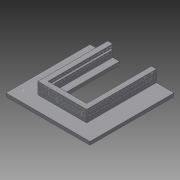
# Autodesk Inventor part: Halterung Merkruphy
Saved by Autodesk Inventor 2015 (Build 190159000, 159)
## iProperties
Created: 2017-01-12
Part Number: Halterung Merkruphy
Material: Generisch
Document SubType Name: Modeling
Designer: nikla
Density: 1 g/cm^3
Appearance: Vorgabe
Author: nikla
Autodesk Inventor part; units mm, degrees
ref_plane "YZ Plane" through (0, 0, 0) normal (1, 0, 0) x (0, 1, 0)
ref_plane "XZ Plane" through (0, 0, 0) normal (0, 1, 0) x (-1, 0, 0)
ref_plane "XY Plane" through (0, 0, 0) normal (0, 0, 1) x (1, 0, 0)
sketch "Skizze4" plane through (0, 0, 0) normal (0, 0, 1) x (1, 0, 0)
  line L0 (0, 0) -> (50, 0)
  line L1 (50, 0) -> (50, 50)
  line L2 (50, 50) -> (0, 50)
  line L3 (0, 50) -> (0, 0)
  dimension "d5" = 50
  dimension "d6" = 50
  constraints: 8 end point, 2 parallel, 1 horizontal, 1 perpendicular
  measures "d5" distance of L2.end L1.end
  measures "d6" distance of L1.end L0.end
extrude "Extrusion1" add sketch "Skizze4" along normal blind 2
sketch "Skizze5" plane through (0, 0, 2) normal (0, 0, 1) x (1, 0, 0)
  line L0 (50, 50) -> (0, 50) projected
  line L1 (17.5, 50) -> (32.5, 50)
  line L2 (32.5, 50) -> (32.5, 12.5)
  line L3 (32.5, 12.5) -> (17.5, 12.5)
  line L4 (17.5, 12.5) -> (17.5, 50)
  point P0 (0, 0)
  dimension "d10" = 15
  dimension "d11" = 37.5
  constraints: 8 end point, 2 parallel, 1 horizontal, 1 perpendicular, 1 point on line
  measures "d10" distance of L2.end L3.end
  measures "d11" distance of L1.end L2.end
extrude "Extrusion2" cut sketch "Skizze5" against normal blind 2
sketch "Skizze6" plane through (0, 0, 2) normal (0, 0, 1) x (1, 0, 0)
  line L0 (17.5, 50) -> (0, 50) projected
  line L1 (12.5, 50) -> (10.5, 50)
  line L2 (10.5, 50) -> (10.5, 10.5)
  line L3 (10.5, 10.5) -> (12.5, 10.5)
  line L4 (12.5, 12.5) -> (12.5, 50)
  line L5 (10.5, 10.5) -> (39.5, 10.5)
  line L6 (39.5, 10.5) -> (39.5, 12.5)
  line L7 (37.5, 12.5) -> (12.5, 12.5)
  line L8 (10.5, 12.5) -> (10.5, 10.5)
  line L9 (50, 50) -> (32.5, 50) projected
  line L10 (39.5, 10.5) -> (37.5, 10.5)
  line L11 (37.5, 12.5) -> (37.5, 50)
  line L12 (37.5, 50) -> (39.5, 50)
  line L13 (39.5, 50) -> (39.5, 10.5)
  point P0 (0, 0)
  dimension "d14" = 2
  dimension "d15" = 39.5
  dimension "d16" = 29
  dimension "d17" = 2
  dimension "d18" = 2
  constraints: 24 end point, 6 parallel, 3 horizontal, 3 perpendicular, 2 point on line
  measures "d14" distance of L3.end L2.end
  measures "d15" distance of L2.end L1.end
  measures "d16" distance of L8.start L6.end
  measures "d17" distance of L6.end L5.end
  measures "d18" distance of L11.end L12.end
extrude "Extrusion3" add sketch "Skizze6" along normal blind 9
sketch "Skizze7" plane through (37.5, 12.5, 2) normal (-1, 0, 0) x (0, 0, 1)
  line L0 (0, -12.5) -> (0, 37.5) projected
  line L1 (9, 37.5) -> (0, 37.5)
  line L2 (0, 37.5) -> (0, 0)
  line L3 (0, 0) -> (9, 0)
  line L4 (9, 0) -> (9, 37.5)
  point P0 (-2, -12.5)
  dimension "d21" = 37.5
  constraints: 8 end point, 2 parallel, 1 horizontal, 1 perpendicular, 1 point on line
  measures "d21" distance of L2.end L1.end
extrude "Extrusion4" add sketch "Skizze7" along normal blind 2
sketch "Skizze9" plane through (35.5, 12.5, 2) normal (-1, 0, 0) x (0, 0, 1)
  line L0 (9, 0) -> (0, 0) projected
  line L1 (7, 37.5) -> (6, 37.5)
  line L2 (6, 37.5) -> (6, 0)
  line L3 (6, 0) -> (7, 0)
  line L4 (7, 0) -> (7, 37.5)
  point P0 (-2, -12.5)
  dimension "d24" = 1
  constraints: 8 end point, 2 parallel, 1 horizontal, 1 perpendicular, 1 point on line
  measures "d24" distance of L3.end L2.end
extrude "Extrusion5" cut sketch "Skizze9" against normal blind 1
sketch "Skizze10" plane through (17.5, 12.5, 0) normal (0, 1, 0) x (1, 0, 0)
  line L0 (18, -2) -> (-5, -2)
  line L1 (-5, -2) -> (-5, -11)
  line L2 (-5, -11) -> (18, -11)
  line L3 (18, -11) -> (18, -2)
  point P0 (-17.5, 0)
  constraints: 8 end point, 2 parallel, 1 horizontal, 1 perpendicular
extrude "Extrusion6" add sketch "Skizze10" along normal blind 2
sketch "Skizze11" plane through (17.5, 14.5, 0) normal (0, 1, 0) x (1, 0, 0)
  line L0 (-5, -11) -> (-5, -2) projected
  line L1 (19, -9) -> (-5, -9)
  line L2 (-5, -9) -> (-5, -8)
  line L3 (-5, -8) -> (19, -8)
  line L4 (19, -8) -> (19, -9)
  point P0 (-17.5, 0)
  constraints: 8 end point, 2 parallel, 1 horizontal, 1 perpendicular, 1 point on line
extrude "Extrusion7" cut sketch "Skizze11" against normal blind 1
sketch "Skizze12" plane through (36.5, 12.5, 9) normal (0, 1, 0) x (1, 0, 0)
  line L0 (-1, 1) -> (0, 1)
  line L1 (0, 1) -> (0, 0)
  line L2 (0, 0) -> (-1, 0)
  line L3 (-1, 0) -> (-1, 1)
  point P0 (-36.5, 9)
  constraints: 8 end point, 2 parallel, 1 horizontal, 1 perpendicular
extrude "Extrusion8" add sketch "Skizze12" along normal blind 1
sketch "Skizze13" plane through (12.5, 50, 11) normal (1, 0, 0) x (0, 0, -1)
  line L0 (9, -35.5) -> (9, -37.5) projected
  line L1 (0, 0) -> (9, 0)
  line L2 (9, 0) -> (9, -36.5)
  line L3 (9, -36.5) -> (0, -36.5)
  line L4 (0, -36.5) -> (0, 0)
  point P0 (11, -50)
  constraints: 8 end point, 2 parallel, 1 horizontal, 1 midpoint, 1 perpendicular
extrude "Extrusion9" add sketch "Skizze13" along normal blind 2
sketch "Skizze14" plane through (14.5, 50, 11) normal (1, 0, 0) x (0, 0, -1)
  line L0 (9, 0) -> (0, 0) projected
  line L1 (2, 0) -> (3, 0)
  line L2 (3, 0) -> (3, -37.5)
  line L3 (3, -37.5) -> (2, -37.5)
  line L4 (2, -37.5) -> (2, 0)
  point P0 (11, -50)
  dimension "d35" = 1
  dimension "d36" = 37.5
  constraints: 8 end point, 2 parallel, 1 horizontal, 1 perpendicular, 1 point on line
  measures "d35" distance of L2.end L3.end
  measures "d36" distance of L1.end L2.end
extrude "Extrusion10" cut sketch "Skizze14" against normal blind 1
sketch "Skizze15" plane through (10.5, 10.5, 2) normal (0, -1, 0) x (1, 0, 0)
  line L0 (0, 9) -> (29, 9)
  line L1 (29, 9) -> (29, 0)
  line L2 (29, 0) -> (0, 0)
  line L3 (0, 0) -> (0, 9)
  point P0 (-10.5, -2)
  constraints: 8 end point, 2 parallel, 1 horizontal, 1 perpendicular
extrude "Extrusion11" add sketch "Skizze15" along normal blind 2
sketch "Skizze16" plane through (17.5, 14.5, 0) normal (0, 1, 0) x (1, 0, 0)
  line L0 (-3, -2) -> (18, -2)
  line L1 (18, -2) -> (18, -8)
  line L2 (18, -8) -> (-3, -8)
  line L3 (-3, -8) -> (-3, -2)
  point P0 (-17.5, 0)
  constraints: 8 end point, 2 parallel, 1 horizontal, 1 perpendicular
extrude "Extrusion12" cut sketch "Skizze16" against normal blind 4
sketch "Skizze17" plane through (17.5, 13.5, 0) normal (0, 1, 0) x (1, 0, 0)
  line L0 (-3, -8) -> (19, -8)
  line L1 (19, -8) -> (19, -9)
  line L2 (19, -9) -> (-3, -9)
  line L3 (-3, -9) -> (-3, -8)
  point P0 (-17.5, 0)
  constraints: 8 end point, 2 parallel, 1 horizontal, 1 perpendicular
extrude "Extrusion13" cut sketch "Skizze17" against normal blind 2
sketch "Skizze18" plane through (14.5, 12.5, 9) normal (0, 1, 0) x (1, 0, 0)
  line L0 (0, 1) -> (-1, 1)
  line L1 (-1, 1) -> (-1, 0)
  line L2 (-1, 0) -> (0, 0)
  line L3 (0, 0) -> (0, 1)
  point P0 (-14.5, 9)
  constraints: 8 end point, 2 parallel, 1 horizontal, 1 perpendicular
extrude "Extrusion14" cut sketch "Skizze18" against normal blind 2
sketch "Skizze19" plane through (17.5, 11.5, 0) normal (0, 1, 0) x (1, 0, 0)
  line L0 (-3, -8) -> (19, -8)
  line L1 (19, -8) -> (19, -9)
  line L2 (19, -9) -> (-3, -9)
  line L3 (-3, -9) -> (-3, -8)
  point P0 (-17.5, 0)
  constraints: 8 end point, 2 parallel, 1 horizontal, 1 perpendicular
extrude "Extrusion15" cut sketch "Skizze19" against normal blind 1
sketch "Skizze20" plane through (36.5, 12.5, 2) normal (-1, 0, 0) x (0, 0, 1)
  line L0 (6, 37.5) -> (7, 37.5)
  line L1 (7, 37.5) -> (7, -2)
  line L2 (7, -2) -> (6, -2)
  line L3 (6, -2) -> (6, 37.5)
  point P0 (-2, -12.5)
  dimension "d49" = 39.5
  constraints: 8 end point, 2 parallel, 1 horizontal, 1 perpendicular
  measures "d49" distance of L0.end L1.end
extrude "Extrusion16" cut sketch "Skizze20" against normal blind 1
sketch "Skizze21" plane through (35.5, 12.5, 2) normal (-1, 0, 0) x (0, 0, 1)
  line L0 (6, 37.5) -> (6, -2) projected
  line L1 (0, 37.5) -> (6, 37.5)
  line L2 (6, 37.5) -> (6, -1)
  line L3 (6, -1) -> (0, -1)
  line L4 (0, -1) -> (0, 37.5)
  point P0 (-2, -12.5)
  dimension "d52" = 38.5
  constraints: 8 end point, 2 parallel, 1 horizontal, 1 perpendicular, 1 point on line
  measures "d52" distance of L1.end L2.end
extrude "Extrusion17" cut sketch "Skizze21" against normal blind 1
sketch "Skizze22" plane through (35.5, 12.5, 2) normal (-1, 0, 0) x (0, 0, 1)
  line L0 (7, 37.5) -> (9, 37.5)
  line L1 (9, 37.5) -> (9, -1)
  line L2 (9, -1) -> (7, -1)
  line L3 (7, -1) -> (7, 37.5)
  point P0 (-2, -12.5)
  dimension "d55" = 38.5
  constraints: 8 end point, 2 parallel, 1 horizontal, 1 perpendicular
  measures "d55" distance of L0.end L1.end
extrude "Extrusion18" cut sketch "Skizze22" against normal blind 1
sketch "Skizze23" plane through (13.5, 50, 11) normal (1, 0, 0) x (0, 0, -1)
  line L0 (2, 0) -> (3, 0)
  line L1 (3, 0) -> (3, -39.5)
  line L2 (3, -39.5) -> (2, -39.5)
  line L3 (2, -39.5) -> (2, 0)
  point P0 (11, -50)
  dimension "d58" = 39.5
  constraints: 8 end point, 2 parallel, 1 horizontal, 1 perpendicular
  measures "d58" distance of L0.end L1.end
extrude "Extrusion19" cut sketch "Skizze23" against normal blind 1
sketch "Skizze24" plane through (14.5, 50, 11) normal (1, 0, 0) x (0, 0, -1)
  line L0 (9, -41.5) -> (9, 0) projected
  line L1 (3, 0) -> (9, 0)
  line L2 (9, 0) -> (9, -38.5)
  line L3 (9, -38.5) -> (3, -38.5)
  line L4 (3, -38.5) -> (3, 0)
  point P0 (11, -50)
  dimension "d62" = 38.5
  constraints: 8 end point, 2 parallel, 1 horizontal, 1 perpendicular, 1 point on line
  measures "d62" distance of L1.end L2.end
extrude "Extrusion20" cut sketch "Skizze24" against normal blind 1
sketch "Skizze25" plane through (14.5, 50, 11) normal (1, 0, 0) x (0, 0, -1)
  line L0 (2, -39.5) -> (2, 0) projected
  line L1 (0, 0) -> (2, 0)
  line L2 (2, 0) -> (2, -38.5)
  line L3 (2, -38.5) -> (0, -38.5)
  line L4 (0, -38.5) -> (0, 0)
  point P0 (11, -50)
  dimension "d65" = 38.5
  constraints: 8 end point, 2 parallel, 1 horizontal, 1 perpendicular, 1 point on line
  measures "d65" distance of L1.end L2.end
extrude "Extrusion21" cut sketch "Skizze25" against normal blind 1
sketch "Skizze26" plane through (17.5, 14.5, 0) normal (0, 1, 0) x (1, 0, 0)
  line L0 (-3, -11) -> (18, -11)
  line L1 (18, -11) -> (18, -9)
  line L2 (18, -9) -> (-3, -9)
  line L3 (-3, -9) -> (-3, -11)
  point P0 (-17.5, 0)
  constraints: 8 end point, 2 parallel, 1 horizontal, 1 perpendicular
extrude "Extrusion22" cut sketch "Skizze26" against normal blind 3
sketch "Skizze27" plane through (14.5, 11.5, 8) normal (0, 1, 0) x (1, 0, 0)
  line L0 (0, 0) -> (-1, 0)
  line L1 (-1, 0) -> (-1, 6)
  line L2 (-1, 6) -> (0, 6)
  line L3 (0, 6) -> (0, 0)
  point P0 (-14.5, 8)
  constraints: 8 end point, 2 parallel, 1 horizontal, 1 perpendicular
extrude "Extrusion23" cut sketch "Skizze27" against normal blind 1
sketch "Skizze28" plane through (35.5, 11.5, 8) normal (0, 1, 0) x (1, 0, 0)
  line L0 (1, 6) -> (0, 6)
  line L1 (0, 6) -> (0, 0)
  line L2 (0, 0) -> (1, 0)
  line L3 (1, 0) -> (1, 6)
  point P0 (-35.5, 8)
  constraints: 8 end point, 2 parallel, 1 horizontal, 1 perpendicular
extrude "Extrusion24" cut sketch "Skizze28" against normal blind 1
sketch "Skizze29" plane through (17.5, 10.5, 0) normal (0, 1, 0) x (1, 0, 0)
  point P0 (-17.5, 0)
sketch "Skizze30" plane through (17.5, 10.5, 0) normal (0, 1, 0) x (1, 0, 0)
  line L0 (19, -8) -> (-4, -8)
  line L1 (-4, -8) -> (-4, -2)
  line L2 (-4, -2) -> (19, -2)
  line L3 (19, -2) -> (19, -8)
  point P0 (-17.5, 0)
  constraints: 8 end point, 2 parallel, 1 horizontal, 1 perpendicular
extrude "Extrusion25" add sketch "Skizze30" along normal blind 1
sketch "Skizze31" plane through (0, 0, 0) normal (0, 0, -1) x (-1, 0, 0)
  line L0 (0, 50) -> (-17.5, 50)
  line L1 (-17.5, 50) -> (-17.5, 12.5)
  line L2 (0, 12.5) -> (0, 50)
  line L3 (-17.5, 12.5) -> (-32.5, 12.5)
  line L4 (-50, 12.5) -> (-50, 0)
  line L5 (-50, 0) -> (0, 0)
  line L6 (0, 0) -> (0, 12.5)
  line L7 (-32.5, 12.5) -> (-32.5, 50)
  line L8 (-32.5, 50) -> (-50, 50)
  line L9 (-50, 50) -> (-50, 12.5)
  constraints: 20 end point, 4 parallel, 2 horizontal, 2 perpendicular, 1 point on line
extrude "Extrusion26" cut sketch "Skizze31" against normal blind 1
sketch "Skizze32" plane through (0, 0, 2) normal (0, 0, 1) x (1, 0, 0)
  line L0 (50, 50) -> (39.5, 50)
  line L1 (39.5, 50) -> (39.5, 8.5)
  line L2 (39.5, 0) -> (50, 0)
  line L3 (50, 0) -> (50, 50)
  line L4 (50, 0) -> (0, 0)
  line L5 (0, 0) -> (0, 8.5)
  line L6 (10.5, 8.5) -> (39.5, 8.5)
  line L7 (50, 8.5) -> (50, 0)
  line L8 (10.5, 8.5) -> (10.5, 50)
  line L9 (10.5, 50) -> (0, 50)
  line L10 (0, 50) -> (0, 8.5)
  constraints: 22 end point, 5 parallel, 2 horizontal, 2 perpendicular
extrude "Extrusion27" add sketch "Skizze32" along normal blind 2
sketch "Skizze33" plane through (0, 0, 2) normal (0, 0, 1) x (1, 0, 0)
  line L0 (17.5, 50) -> (17.5, 12.5)
  line L1 (17.5, 12.5) -> (32.5, 12.5)
  line L2 (32.5, 12.5) -> (32.5, 50)
  line L3 (32.5, 50) -> (32.5, 12.5) projected
  line L4 (32.5, 50) -> (36.5, 50)
  line L5 (36.5, 50) -> (36.5, 11.5)
  line L6 (36.5, 11.5) -> (36.5, 50) projected
  line L7 (36.5, 11.5) -> (13.5, 11.5)
  line L8 (13.5, 11.5) -> (13.5, 50)
  line L9 (17.5, 50) -> (13.5, 50) projected
  line L10 (13.5, 50) -> (17.5, 50)
  point P0 (0, 0)
  constraints: 16 end point, 5 perpendicular, 2 collinear, 1 vertical
extrude "Extrusion28" add sketch "Skizze33" along normal blind 2 and the other way blind 1
sketch "Skizze34" plane through (0, 0, 1) normal (0, 0, -1) x (-1, 0, 0)
  line L0 (-32.5, 50) -> (-50, 50)
  line L1 (-50, 50) -> (-50, 0)
  line L2 (-50, 0) -> (0, 0)
  line L3 (0, 0) -> (0, 50)
  line L4 (0, 50) -> (-17.5, 50)
  line L5 (-17.5, 50) -> (-17.5, 12.5)
  line L6 (-17.5, 12.5) -> (-32.5, 12.5)
  line L7 (-32.5, 12.5) -> (-32.5, 50)
  constraints: 16 end point, 7 perpendicular, 1 horizontal
extrude "Extrusion29" cut sketch "Skizze34" against normal blind 1
